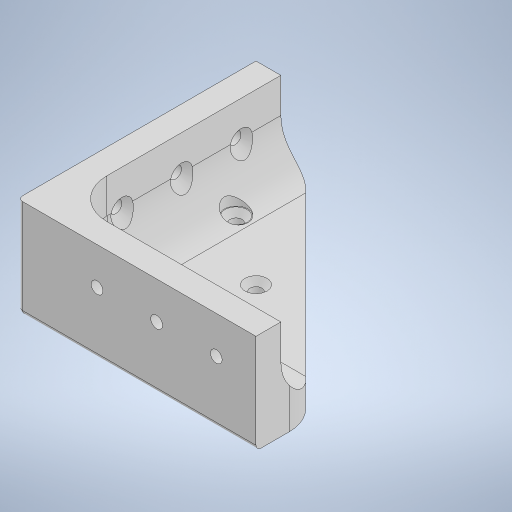
# Autodesk Inventor part: Arena Tri Corner Bracket
Saved by Autodesk Inventor 2023.4 (Build 274418000, 418)
## iProperties
Created: 2024-04-25
Part Number: Arena Tri Corner Bracket
Material: Generic
Document SubType Name: Modeling
Designer: Nathan Cai
Density: 1 g/cm^3
Appearance: Default
Author: Nathan Cai
Autodesk Inventor part; units mm, degrees
ref_plane "YZ Plane" through (0, 0, 0) normal (1, 0, 0) x (0, 1, 0)
ref_plane "XZ Plane" through (0, 0, 0) normal (0, 1, 0) x (-1, 0, 0)
sketch "Sketch1" plane through (0, 0, 0) normal (0, 1, 0) x (-1, 0, 0)
  line L0 (-38.1, 38.1) -> (38.1, 38.1)
  line L1 (38.1, 38.1) -> (38.1, -38.1)
  line L2 (38.1, -38.1) -> (-38.1, -38.1)
  line L3 (-38.1, -38.1) -> (-38.1, 38.1)
  line L4 (-38.1, 38.1) -> (38.1, -38.1) construction
  line L5 (38.1, 38.1) -> (-38.1, -38.1) construction
  line L6 (38.1, 38.1) -> (30.1625, 38.1)
  line L7 (30.1625, 38.1) -> (30.1625, -38.1)
  line L8 (30.1625, -38.1) -> (38.1, -38.1)
  line L9 (38.1, -38.1) -> (38.1, 38.1)
  line L10 (38.1, 38.1) -> (-38.1, 38.1)
  line L11 (-38.1, 38.1) -> (-38.1, 30.1625)
  line L12 (-38.1, 30.1625) -> (38.1, 30.1625)
  line L13 (38.1, 30.1625) -> (38.1, 38.1)
  line L14 (-38.1, 22.225) -> (22.225, -38.1)
  point P0 (0, 0)
  point P1 (30.1625, 30.1625)
  dimension "d0" = 76.2
  dimension "d1" = 76.2
  dimension "d2" = 7.9375
  dimension "d3" = 7.9375
  dimension "d6" = 7.9375
  dimension "d7" = 7.9375
  constraints: 30 end point, 6 parallel, 4 point on line, 3 horizontal, 3 perpendicular, 2 midpoint
  measures "d0" distance of L1.end L2.end
  measures "d1" distance of L0.end L1.end
  measures "d2" distance of L8.end L7.end
  measures "d3" distance of L11.end L10.end
  measures "d6" distance of L14.end L7.end
  measures "d7" distance of L11.end L14.start
extrude "Extrusion1" add sketch "Sketch1" along normal blind 7.9375 contours L0 L7 L12 L3 | L0 L1 L12 L7 | L12 L7 L2 L14 L3 | L12 L1 L2 L7
extrude "Extrusion2" add sketch "Sketch1" along normal blind 31.75 contours L0 L7 L12 L3 | L0 L1 L12 L7 | L12 L1 L2 L7
sketch "Sketch2" plane through (-30.1625, 0, -38.1) normal (-1, 0, 0) x (0, 0, 1)
  line L0 (0, 7.9375) -> (0, 31.75) projected
  line L1 (0, 19.8437) -> (76.2, 19.8438) construction
  line L2 (76.2, 0) -> (76.2, 31.75) projected
  point P0 (38.1, 0)
  point P1 (12.7, 19.8438)
  point P2 (31.75, 19.8438)
  point P3 (50.8, 19.8438)
  dimension "d11" = 12.7
  dimension "d14" = 19.05
  constraints: 2 end point, 2 horizontal, 2 point on line, 1 midpoint, 2 other
  measures "d11" distance from line of L0 point (12.7, 19.844)
  measures "d14" distance of point (12.7, 19.844) point (31.75, 19.844)
ref_plane "Work Plane1" through (-30.1625, 7.9375, 30.1625) normal (-0.7071068, 0, -0.7071068) x (0, 1, 0)
hole "Hole1" at (-30.1625, 19.8438, -25.4) at (-30.1625, 19.8438, -6.35) at (-30.1625, 19.8438, 12.7) direction (-1, 0, 0) diameter 3.81 end through all countersink diameter 7.0866 countersink angle 82 clearance for "Flat Head Machine Screw (82)" size "#6" standard "Ansi Unified Screw Threads"
mirror "Mirror1" about plane through (-30.1625, 7.9375, 30.1625) normal (-0.7071068, 0, -0.7071068) of "Hole1"
fillet "Fillet1" radius 12.7 5 edges at (-30.1625, 19.8438, 30.1625) (-30.1625, 7.9375, -3.9688) (3.9687, 7.9375, 30.1625) (38.1, 3.9688, 22.225) (-22.225, 3.9688, -38.1)
sketch "Sketch3" plane through (0, 7.9375, 0) normal (0, 1, 0) x (1, 0, 0)
  line L0 (-22.225, 38.1) -> (-30.1625, 38.1) projected
  line L1 (-22.225, 38.1) -> (-22.225, -30.1625) construction
  line L2 (-30.1625, -30.1625) -> (38.1, -30.1625) projected
  line L3 (38.1, -22.225) -> (-22.225, 38.1) projected
  line L4 (38.1, -22.225) -> (-30.1625, -22.225) construction
  line L5 (-30.1625, -30.1625) -> (-30.1625, 38.1) projected
  point P0 (0, 0)
  point P1 (-22.225, -22.225)
  point P2 (0, 0)
  point P3 (-22.225, 15.875)
  point P4 (15.875, -22.225)
  point P5 (15.875, 15.875)
  dimension "d28" = 38.1
  dimension "d31" = 38.1
  constraints: 4 end point, 4 point on line, 2 vertical, 1 coincident, 1 horizontal, 1 perpendicular, 3 other
  measures "d28" distance of point (-22.225, -22.225) point (-22.225, 15.875)
  measures "d31" distance of point (-22.225, -22.225) point (15.875, -22.225)
hole "Hole2" at (-22.225, 7.9375, 22.225) at (0, 7.9375, 0) at (-22.225, 7.9375, -15.875) at (15.875, 7.9375, 22.225) at (15.875, 7.9375, -15.875) direction (0, -1, 0) diameter 3.81 end through all countersink diameter 7.0866 countersink angle 82 clearance for "Flat Head Machine Screw (82)" size "#6" standard "Ansi Unified Screw Threads"
fillet "Fillet2" radius 1.5875 3 edges at (-38.1, 15.875, 38.1) (0, 0, 38.1) (-38.1, 0, 0)
hole "Hole3" at (15.875, 7.9375, 22.225) at (-22.225, 7.9375, -15.875) at (0, 7.9375, 0) at (-22.225, 7.9375, 22.225) direction (0, 1, 0) diameter 7.62 end through all
equation "\"d6\" = d2"
equation "\"d7\" = d3"
body "Solid1"
